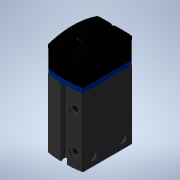
# Autodesk Inventor part: 1310162 DHRS-25-A---(Geh)
Saved by Autodesk Inventor 2021 (Build 250183000, 183)
## iProperties
Created: 2026-04-25
Part Number: 1310162 DHRS-25-A---(Geh)
Material: Generic
Catalog Web Link: www.3dfindit.com
Description: DHRS---(Geh)-Housing
Vendor: FESTO
Document SubType Name: Modeling
Designer: psAdmin
Manufacturer: FESTO
Mass: 95.5406 g
Surface Area: 179.925 cm^2
Volume: 95.5406 cm^3
Density: 1 g/cm^3
Appearance: PSOLRGB-176-176-176
Category: PARTsolutions
Company: FESTO
Title: 1310162 DHRS-25-A---(Geh)
Author: Cadenas PARTsolutions
Comments: Housing
PSOL_IDENT_0: {$CADENAS_DATA/23d-libs/festo/parts/d/dhrs/parts/dhrs_geh.prj},196 {VTYP=3D},{NB=1310162 DHRS-25-A--
PSOL_IDENT_1: -(Geh)},{LINA=1310162 DHRS-25-A---(Geh)},{NN=DHRS---(Geh)},{DATE=17.04.2026 13:59:02},{GEOMDATE=22.0
PSOL_IDENT_2: 8.2023 11:13:58},{VERSION=},{LINEID=40},{WBVAR=},{WBNUMERIC=}  {NB=1310162 DHRS-25-A---(Geh)},{LINA=
PSOL_IDENT_3: 1310162 DHRS-25-A---(Geh)},{KT=DUMMY},{TNR=1310162},{TYP=DHRS-25-A},{GR=25}
NB: 1310162 DHRS-25-A---(Geh)
NN: DHRS---(Geh)
NT: Housing
NBSYN: $TNR. $TYP.---(Geh)
LINA: 1310162 DHRS-25-A---(Geh)
CATALOG: Festo
TNR: 1310162
TYP: DHRS-25-A
GR: 25
SUPPLIER: FESTO
ARTICLENO: 1310162 DHRS-25-A---(Geh)
BOMINFO: 1310162 DHRS-25-A---(Geh)
CREATOR: CADENAS GmbH
Autodesk Inventor part; units mm, degrees
sketch "Sketch_1" plane through (0, 0, 0) normal (0, 1, 0) x (-1, 0, 0)
  line L0 (14.75, -20.1685) -> (14.75, 20.1685)
  arc A0 (14.75, 20.1685) -> (14.162, 20.8595) centre (14.05, 20.1685) ccw
  arc A1 (14.162, 20.8595) -> (2.6, 21.9618) centre (0, -66.5) ccw
  line L1 (2.6, 21.9618) -> (2.6, 20.4)
  line L2 (2.6, 20.4) -> (3.25, 20.4)
  line L3 (3.25, 20.4) -> (3.25, 17.2)
  line L4 (3.25, 17.2) -> (-3.25, 17.2)
  line L5 (-3.25, 17.2) -> (-3.25, 20.4)
  line L6 (-3.25, 20.4) -> (-2.6, 20.4)
  line L7 (-2.6, 20.4) -> (-2.6, 21.9618)
  arc A2 (-2.6, 21.9618) -> (-14.162, 20.8595) centre (0, -66.5) ccw
  arc A3 (-14.162, 20.8595) -> (-14.75, 20.1685) centre (-14.05, 20.1685) ccw
  line L8 (-14.75, 20.1685) -> (-14.75, -20.1685)
  arc A4 (-14.75, -20.1685) -> (-14.162, -20.8595) centre (-14.05, -20.1685) ccw
  arc A5 (-14.162, -20.8595) -> (-2.6, -21.9618) centre (0, 66.5) ccw
  line L9 (-2.6, -21.9618) -> (-2.6, -20.4)
  line L10 (-2.6, -20.4) -> (-3.25, -20.4)
  line L11 (-3.25, -20.4) -> (-3.25, -17.2)
  line L12 (-3.25, -17.2) -> (3.25, -17.2)
  line L13 (3.25, -17.2) -> (3.25, -20.4)
  line L14 (3.25, -20.4) -> (2.6, -20.4)
  line L15 (2.6, -20.4) -> (2.6, -21.9618)
  arc A6 (2.6, -21.9618) -> (14.162, -20.8595) centre (0, 66.5) ccw
  arc A7 (14.162, -20.8595) -> (14.75, -20.1685) centre (14.05, -20.1685) ccw
  constraints: 32 end point, 16 point on circle, 8 centre point
extrude "Extrusion1" add sketch "Sketch_1" along normal blind 57
sketch "Sketch_2" plane through (0, 61, 0) normal (0, 1, 0) x (1, 0, 0)
  line L0 (-14.655, 20.0725) -> (-14.655, -20.0725)
  arc A0 (-14.655, -20.0725) -> (-14.0664, -20.7636) centre (-13.955, -20.0725) ccw
  arc A1 (-14.0664, -20.7636) -> (14.0664, -20.7636) centre (0, 66.5) ccw
  arc A2 (14.0664, -20.7636) -> (14.655, -20.0725) centre (13.955, -20.0725) ccw
  line L1 (14.655, -20.0725) -> (14.655, 20.0725)
  arc A3 (14.655, 20.0725) -> (14.0664, 20.7636) centre (13.955, 20.0725) ccw
  arc A4 (14.0664, 20.7636) -> (-14.0664, 20.7636) centre (0, -66.5) ccw
  arc A5 (-14.0664, 20.7636) -> (-14.655, 20.0725) centre (-13.955, 20.0725) ccw
  constraints: 12 point on circle, 6 centre point, 4 end point
extrude "Extrusion2" add sketch "Sketch_2" against normal blind 4
sketch "Sketch_3" plane through (0, 61, 0) normal (0, 1, 0) x (1, 0, 0)
  line L0 (-14.675, 20.0996) -> (-14.675, -20.0996)
  arc A0 (-14.675, -20.0996) -> (-14.0865, -20.7907) centre (-13.975, -20.0996) ccw
  arc A1 (-14.0865, -20.7907) -> (14.0865, -20.7907) centre (0, 66.5) ccw
  arc A2 (14.0865, -20.7907) -> (14.675, -20.0996) centre (13.975, -20.0996) ccw
  line L1 (14.675, -20.0996) -> (14.675, 20.0996)
  arc A3 (14.675, 20.0996) -> (14.0865, 20.7907) centre (13.975, 20.0996) ccw
  arc A4 (14.0865, 20.7907) -> (-14.0865, 20.7907) centre (0, -66.5) ccw
  arc A5 (-14.0865, 20.7907) -> (-14.675, 20.0996) centre (-13.975, 20.0996) ccw
  constraints: 12 point on circle, 6 centre point, 4 end point
extrude "Extrusion3" add sketch "Sketch_3" along normal blind 25
sketch "Sketch_4" plane through (0, 0, 0) normal (0, 0, 1) x (1, 0, 0)
  line L0 (10, 18.1) -> (-10, 18.1)
  arc A0 (20, 79.2223) -> (-20, 79.2223) centre (0, 39.75) ccw
  line L1 (20, 79.2223) -> (20, 95)
  line L2 (20, 95) -> (-20, 95)
  line L3 (-20, 95) -> (-20, 79.2223)
  constraints: 8 end point, 2 point on circle, 1 centre point
revolve "Revolution1" cut sketch "Sketch_4" angle 60 mid plane about axis through (10, 18.1, 0) along (-1, 0, 0)
sketch "Sketch_5" plane through (0, 0, 0) normal (1, 0, 0) x (0, 1, 0)
  line L0 (73.5263, 26.91) -> (73.5263, 21.91)
  arc A0 (82.2917, 14.9516) -> (73.5263, 21.91) centre (73.5263, 12.91) ccw
  arc A1 (82.2917, -14.9516) -> (82.2917, 14.9516) centre (18.1, 0) ccw
  arc A2 (73.5263, -21.91) -> (82.2917, -14.9516) centre (73.5263, -12.91) ccw
  line L1 (73.5263, -21.91) -> (73.5263, -26.91)
  line L2 (73.5263, -26.91) -> (90, -26.91)
  line L3 (90, -26.91) -> (90, 26.91)
  line L4 (90, 26.91) -> (73.5263, 26.91)
  constraints: 10 end point, 6 point on circle, 3 centre point
extrude "Extrusion4" cut sketch "Sketch_5" along normal mid plane 40
sketch "Sketch_7" plane through (0, 65.5, 0) normal (0, 1, 0) x (1, 0, 0)
  line L0 (-2.5, -9.275) -> (-2.5, -25)
  line L1 (-2.5, -25) -> (2.5, -25)
  line L2 (2.5, -25) -> (2.5, -9.275)
  arc A0 (-2.5, -9.275) -> (2.5, -9.275) centre (0, 4.5) ccw
  constraints: 6 end point, 2 point on circle, 1 centre point
extrude "Extrusion5" cut sketch "Sketch_7" along normal blind 20
sketch "Sketch_19" plane through (0, 65.5, 0) normal (0, 1, 0) x (1, 0, 0)
  arc A0 (2.5, 9.275) -> (-2.5, 9.275) centre (0, -4.5) ccw
  line L0 (2.5, 9.275) -> (2.5, 25)
  line L1 (2.5, 25) -> (-2.5, 25)
  line L2 (-2.5, 25) -> (-2.5, 9.275)
  constraints: 6 end point, 2 point on circle, 1 centre point
extrude "Extrusion6" cut sketch "Sketch_19" along normal blind 20
sketch "Sketch_6" plane through (0, 0, 0) normal (1, 0, 0) x (0, 1, 0)
  circle A0 centre (72, 11.1) radius 10.9
  constraints: 1 centre point
extrude "Extrusion7" cut sketch "Sketch_6" along normal mid plane 5
sketch "Sketch_17" plane through (0, 0, 0) normal (1, 0, 0) x (0, 1, 0)
  circle A0 centre (72, -11.1) radius 10.9
  constraints: 1 centre point
extrude "Extrusion8" cut sketch "Sketch_17" along normal mid plane 5
sketch "Sketch_10" plane through (0, 0, 21) normal (0, 0, 1) x (1, 0, 0)
  arc A0 (8.75, 47.3) -> (8.75, 38.3) centre (8.75, 42.8) ccw
  line L0 (8.75, 38.3) -> (18.75, 38.3)
  line L1 (18.75, 38.3) -> (18.75, 16.3)
  line L2 (18.75, 16.3) -> (8.75, 16.3)
  arc A1 (8.75, 16.3) -> (8.75, 7.3) centre (8.75, 11.8) ccw
  line L3 (8.75, 7.3) -> (23.75, 7.3)
  line L4 (23.75, 7.3) -> (23.75, 47.3)
  line L5 (23.75, 47.3) -> (8.75, 47.3)
  constraints: 12 end point, 4 point on circle, 2 centre point
extrude "Extrusion9" cut sketch "Sketch_10" along normal blind 3
sketch "Sketch11" plane through (0, 0, 21) normal (0, 0, 1) x (1, 0, 0)
  point P0 (8.75, 11.8)
hole "Hole1" at (8.75, 11.8, 21) direction (0, 0, -1) diameter 4.134 depth 6.5 countersink diameter 5 countersink angle 90 thread size "M5x0.8" class "6H" standard "ISO Metric profile"
sketch "Sketch12" plane through (0, 0, 21) normal (0, 0, 1) x (1, 0, 0)
  point P0 (8.75, 42.8)
hole "Hole2" at (8.75, 42.8, 21) direction (0, 0, -1) diameter 4.134 depth 6.5 countersink diameter 5 countersink angle 90 thread size "M5x0.8" class "6H" standard "ISO Metric profile"
sketch "Sketch13" plane through (-14.75, 0, -20.1685) normal (-1, 0, 0) x (0, 0, 1)
  point P0 (32.6685, 7.5)
hole "Hole3" at (-14.75, 7.5, 12.5) direction (1, 0, 0) diameter 3.242 depth 14.75 counterbore diameter 7 counterbore depth 1.6 thread size "M4x0.7" class "6H" standard "ISO Metric profile"
sketch "Sketch14" plane through (14.75, 0, 20.1685) normal (1, 0, 0) x (0, 0, -1)
  point P0 (7.6685, 7.5)
hole "Hole4" at (14.75, 7.5, 12.5) direction (-1, 0, 0) diameter 3.242 depth 14.75 counterbore diameter 7 counterbore depth 1.6 thread size "M4x0.7" class "6H" standard "ISO Metric profile"
sketch "Sketch15" plane through (-14.75, 0, -20.1685) normal (-1, 0, 0) x (0, 0, 1)
  point P0 (7.6685, 7.5)
hole "Hole5" at (-14.75, 7.5, -12.5) direction (1, 0, 0) diameter 3.242 depth 14.75 counterbore diameter 7 counterbore depth 1.6 thread size "M4x0.7" class "6H" standard "ISO Metric profile"
sketch "Sketch16" plane through (14.75, 0, 20.1685) normal (1, 0, 0) x (0, 0, -1)
  point P0 (32.6685, 7.5)
hole "Hole6" at (14.75, 7.5, -12.5) direction (-1, 0, 0) diameter 3.242 depth 14.75 counterbore diameter 7 counterbore depth 1.6 thread size "M4x0.7" class "6H" standard "ISO Metric profile"
sketch "Sketch17" plane through (0, 0, 0) normal (0, -1, 0) x (1, 0, 0)
  point P0 (0, 12.5)
hole "Hole7" at (0, 0, 12.5) direction (0, 1, 0) diameter 3.242 depth 7.5 counterbore diameter 7 counterbore depth 1.6 thread size "M4x0.7" class "6H" standard "ISO Metric profile"
sketch "Sketch18" plane through (0, 0, 0) normal (0, -1, 0) x (1, 0, 0)
  point P0 (0, -12.5)
hole "Hole8" at (0, 0, -12.5) direction (0, 1, 0) diameter 3.242 depth 7.5 counterbore diameter 7 counterbore depth 1.6 thread size "M4x0.7" class "6H" standard "ISO Metric profile"
sketch "Sketch_22" plane through (0, 0, 0) normal (1, 0, 0) x (0, 1, 0)
  arc A0 (62.1345, 17.7544) -> (66.5975, 0.497) centre (72, 11.1) ccw
  line L0 (66.5975, 0.497) -> (72, 11.1)
  line L1 (72, 11.1) -> (62.1345, 17.7544)
  constraints: 4 end point, 2 point on circle, 1 centre point
extrude "Extrusion10" cut sketch "Sketch_22" along normal mid plane 1.5
sketch "Sketch_23" plane through (0, 0, 0) normal (1, 0, 0) x (0, 1, 0)
  arc A0 (66.5975, -0.497) -> (62.1345, -17.7544) centre (72, -11.1) ccw
  line L0 (62.1345, -17.7544) -> (72, -11.1)
  line L1 (72, -11.1) -> (66.5975, -0.497)
  constraints: 4 end point, 2 point on circle, 1 centre point
extrude "Extrusion11" cut sketch "Sketch_23" along normal mid plane 1.5
ref_plane "GEHAEUSE_XY" through (0, 0, 0) normal (0, 1, 0) x (1, 0, 0)
ref_plane "GEHAEUSE_YZ" through (0, 0, 0) normal (1, 0, 0) x (0, 0, -1)
ref_plane "GEHAEUSE_ZX" through (0, 0, 0) normal (0, 0, -1) x (0, 1, 0)
ref_plane "TO_JAW_L_XY" through (0, 72, 11.1) normal (1, 0, 0) x (0, 0, -1)
ref_plane "TO_JAW_L_YZ" through (0, 72, 11.1) normal (0, 0, -1) x (0, 1, 0)
ref_plane "TO_JAW_L_ZX" through (0, 72, 11.1) normal (0, 1, 0) x (1, 0, 0)
ref_plane "TO_JAW_R_XY" through (0, 72, -11.1) normal (1, 0, 0) x (0, 0, -1)
ref_plane "TO_JAW_R_YZ" through (0, 72, -11.1) normal (0, 0, -1) x (0, 1, 0)
ref_plane "TO_JAW_R_ZX" through (0, 72, -11.1) normal (0, 1, 0) x (1, 0, 0)
ref_plane "TO_ZBH_1_XY" through (0, 1.6, -12.5) normal (0, 1, 0) x (1, 0, 0)
ref_plane "TO_ZBH_1_YZ" through (0, 1.6, -12.5) normal (1, 0, 0) x (0, 0, -1)
ref_plane "TO_ZBH_1_ZX" through (0, 1.6, -12.5) normal (0, 0, -1) x (0, 1, 0)
ref_plane "TO_ZBH_2_XY" through (0, 1.6, 12.5) normal (0, 1, 0) x (1, 0, 0)
ref_plane "TO_ZBH_2_YZ" through (0, 1.6, 12.5) normal (1, 0, 0) x (0, 0, -1)
ref_plane "TO_ZBH_2_ZX" through (0, 1.6, 12.5) normal (0, 0, -1) x (0, 1, 0)
body "Solid1"
